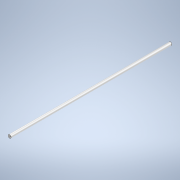
# Autodesk Inventor part: barra
Saved by Autodesk Inventor 2021 (Build 250183000, 183)
## iProperties
Created: 2021-04-15
Part Number: barra
Material: Acero inoxidable AISI 304
Document SubType Name: Modeling
Designer: leo7s
Density: 8 g/cm^3
Appearance: Cromo - Satinado
Mass: 1296.85 g
Surface Area: 412.417 cm^2
Volume: 162.107 cm^3
Author: leo7s
Autodesk Inventor part; units mm, degrees
ref_plane "YZ Plane" through (0, 0, 0) normal (1, 0, 0) x (0, 1, 0)
ref_plane "XZ Plane" through (0, 0, 0) normal (0, 1, 0) x (-1, 0, 0)
ref_plane "XY Plane" through (0, 0, 0) normal (0, 0, 1) x (1, 0, 0)
sketch "Boceto2" plane through (0, 0, 0) normal (0, 0, 1) x (1, 0, 0)
  circle A0 centre (0, 0) radius 7.9375
  dimension "d0" = 15.875
  constraints: 1 centre point, 1 coincident
  measures "d0" diameter of A0
extrude "Extrusión1" add sketch "Boceto2" against normal blind 815
sketch "Boceto3" plane through (0, 0, 0) normal (0, 0, 1) x (1, 0, 0)
  circle A0 centre (0, 0) radius 7.9375 projected
extrude "Extrusión2" add sketch "Boceto3" along normal blind 4
sketch "Boceto4" plane through (0, 0, 4) normal (0, 0, 1) x (1, 0, 0)
  circle A0 centre (0, 0) radius 3.175
  dimension "d5" = 6.35
  constraints: 1 centre point, 1 coincident
  measures "d5" diameter of A0
extrude "Extrusión3" cut sketch "Boceto4" against normal blind 38.1
thread "Rosca1" size "1/4-20 UNC" class "1B" standard "ANSI Unified Screw Threads" length 30
sketch "Boceto5" plane through (0, 0, -815) normal (0, 0, -1) x (-1, 0, 0)
  circle A0 centre (0, 0) radius 3.175
  dimension "d10" = 6.35
  constraints: 1 centre point, 1 coincident
  measures "d10" diameter of A0
extrude "Extrusión4" cut sketch "Boceto5" against normal blind 38.1
thread "Rosca2" size "1/4-20 UNC" class "1B" standard "ANSI Unified Screw Threads" length 30
